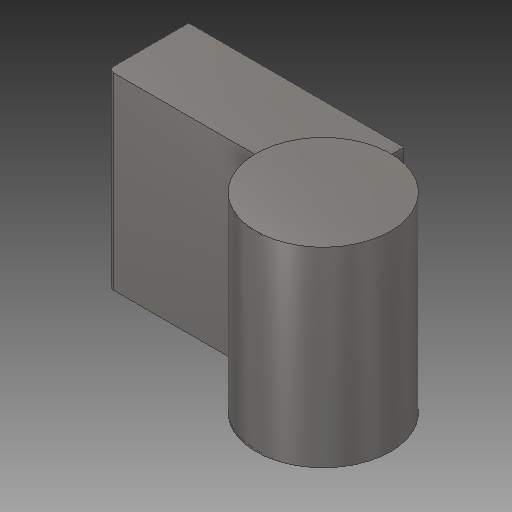
# Autodesk Inventor part: Battery Box
Saved by Autodesk Inventor 2019 (Build 230136000, 136)
## iProperties
Created: 2019-08-29
Part Number: Battery Box
Material: Steel, Mild
Document SubType Name: Sheet Metal
Designer: DIBYOJYOTI
Density: 7.85 g/cm^3
Sheet Metal Rule: Default
Appearance: Semi-Polished
Mass: 84.0893 g
Surface Area: 444.693 cm^2
Volume: 10.712 cm^3
Author: DIBYOJYOTI
Autodesk Inventor part; units mm, degrees
ref_plane "YZ Plane" through (0, 0, 0) normal (1, 0, 0) x (0, 1, 0)
ref_plane "XZ Plane" through (0, 0, 0) normal (0, 1, 0) x (-1, 0, 0)
ref_plane "XY Plane" through (0, 0, 0) normal (0, 0, 1) x (1, 0, 0)
sketch "Sketch1" plane through (0, 0, 0) normal (0, 0, 1) x (1, 0, 0)
  line L0 (-40, 35) -> (40, 35)
  line L1 (40, 35) -> (40, -35)
  line L2 (40, -35) -> (-40, -35)
  line L3 (-40, -35) -> (-40, 35)
  line L4 (-40, 35) -> (40, -35) construction
  line L5 (40, 35) -> (-40, -35) construction
  point P0 (0, 0)
  dimension "d0" = 70
  dimension "d1" = 80
  constraints: 12 end point, 2 midpoint, 2 parallel, 1 horizontal, 1 perpendicular
  measures "d0" distance of L0.end L1.end
  measures "d1" distance of L1.end L2.end
extrude "Extrusion1" add sketch "Sketch1" along normal blind 30
sketch "Sketch2" plane through (-40, 35, 0) normal (0, 1, 0) x (1, 0, 0)
  line L0 (80, -30) -> (0, -30) projected
  circle A0 centre (80, -30) radius 25
  point P0 (40, 0)
  dimension "d4" = 50
  constraints: 1 centre point
  measures "d4" diameter of A0
extrude "Extrusion2" add sketch "Sketch2" against normal blind 70
extrude "Extrusion3" add sketch "Sketch2" along normal blind 0.5
sketch "Sketch3" plane through (-40, -35, 0) normal (0, -1, 0) x (1, 0, 0)
  circle A0 centre (79.901, 30.2944) radius 25
  line L0 (53.0517, 30.2944) -> (54.901, 30.2944)
  circle A1 centre (79.901, 30.2944) radius 24.5
  point P0 (40, 0)
  dimension "d9" = 50
  dimension "d19" = 49
  constraints: 2 end point, 1 centre point, 1 coincident, 1 horizontal, 1 horizontal alignment, 2 other
  measures "d19" diameter of A1
fillet "Fillet1" radius 2 1 edges at (-40, 0, 30)
sketch "Sketch4" plane through (0, 0, 0) normal (0, 0, -1) x (-1, 0, 0)
  line L0 (40, -35) -> (38, -35) projected
  line L1 (40, -35) -> (39, -35)
  line L2 (-40, 35) -> (-15, 35) projected
  line L3 (-40, 35) -> (-39, 35)
  line L4 (39.5, -34.5) -> (-39.5, -34.5)
  line L5 (-39.5, -34.5) -> (-39.5, 34.5)
  line L6 (-39.5, 34.5) -> (39.5, 34.5)
  line L7 (39.5, 34.5) -> (39.5, -34.5)
  line L8 (40, -35) -> (40, 35) projected
  line L9 (-40, 35) -> (-40, -35) projected
  line L10 (-40, -35) -> (40, -35) projected
  line L11 (40, 35) -> (-40, 35) projected
  point P0 (0, 0)
  dimension "d24" = 0.5
  dimension "d25" = 0.5
  dimension "d26" = 0.5
  dimension "d27" = 0.5
  constraints: 12 end point, 3 horizontal, 2 parallel, 1 perpendicular
  measures "d24" distance between parallel lines of L8 L7
  measures "d25" distance between parallel lines of L9 L5
  measures "d26" distance between parallel lines of L10 L4
  measures "d27" distance between parallel lines of L11 L6
extrude "Extrusion6" cut sketch "Sketch3" against normal blind 70 contours A1
sketch "Sketch5" plane through (-40, -35, 0) normal (0, -1, 0) x (1, 0, 0)
  arc A0 (80, 5) -> (55, 30) centre (80, 30) ccw projected
  circle A1 centre (80, 30) radius 25
  point P0 (40, 0)
  constraints: 1 centre point, 1 coincident
extrude "Extrusion7" add sketch "Sketch5" along normal blind 0.5
extrude "Extrusion8" cut sketch "Sketch4" against normal blind 29.5 contours L4 L5 L6 L7
equation "\"BendRadius\" = Thickness"
equation "\"BendReliefWidth\" = Thickness"
equation "\"BendReliefDepth\" = 0.5 * Thickness"
equation "\"CornerReliefSize\" = 4 * Thickness"
equation "\"MinimumRemnant\" = 2 * Thickness"
equation "\"TransitionRadius\" = BendRadius"
equation "\"JacobiRadiusSize\" = Thickness"
equation "\"GapSize\" = Thickness"
equation "\"Thickness\" = 0.5"
body "Solid1"
